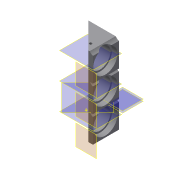
# Autodesk Inventor part: 30_Cube_Insert_Filter_Revolver_Filter_base
Saved by Autodesk Inventor 2019.4 (Build 234330000, 330)
## iProperties
Created: 2021-09-13
Part Number: 30_Cube_Insert_Filter_Revolver_Filter_base
Material: Generic
Document SubType Name: Modeling
Designer: diederichbenedict
Density: 1 g/cm^3
Appearance: Default
Mass: 6.97028 g
Surface Area: 48.8121 cm^2
Volume: 6.97028 cm^3
Author: diederichbenedict
Autodesk Inventor part; units mm, degrees
ref_plane "YZ Plane" through (0, 0, 0) normal (1, 0, 0) x (0, 1, 0)
ref_plane "XZ Plane" through (0, 0, 0) normal (0, 1, 0) x (-1, 0, 0)
ref_plane "XY Plane" through (0, 0, 0) normal (0, 0, 1) x (1, 0, 0)
ref_plane "Work Plane1" through (-34.3358, -34.38, 2.0699) normal (0, -1, 0) x (0.7071068, 0, -0.7071068)
ref_plane "Work Plane4" through (-9.5871, -34.38, 28.2329) normal (0, -1, 0) x (1, 0, 0)
ref_plane "Work Plane3" through (-9.5871, -32.38, 28.2329) normal (0, -1, 0) x (1, 0, 0)
sketch "Sketch1" plane through (-9.5871, -34.38, 28.2329) normal (0, -1, 0) x (1, 0, 0)
  line L0 (0.7071, -1.3185) -> (0.7071, -26.3185) construction
  line L1 (0.7071, -1.3185) -> (1.7071, -1.3185) construction
  line L2 (0.7071, -26.3185) -> (1.7071, -26.3185) construction
  line L3 (0.7071, -0.7071) -> (-26.8187, -28.2329)
  line L4 (-26.8187, -28.2329) -> (0.7071, -28.2329)
  line L5 (0.7071, -28.2329) -> (0.7071, -0.7071)
  line L6 (0.7071, -0.7071) -> (5.7071, -0.7071)
  line L7 (5.7071, -0.7071) -> (5.7071, -28.2329)
  line L8 (5.7071, -28.2329) -> (0.7071, -28.2329)
  line L9 (0.7071, -0.7071) -> (5.7071, -0.7071)
  line L10 (5.7071, -0.7071) -> (5.7071, 1.3671)
  line L11 (5.7071, 1.3671) -> (0.7071, 1.3671)
  line L12 (0.7071, 1.3671) -> (0.7071, -0.7071)
  line L13 (2.5336, 1.8671) -> (2.3871, 1.8671) projected
  line L14 (0.7071, -0.7071) -> (0.7071, -28.2329)
  line L15 (0.7071, -28.2329) -> (-26.8187, -28.2329)
  line L16 (-26.8187, -28.2329) -> (0.7071, -0.7071)
  point P0 (9.5871, -28.2329)
  dimension "d1" = 5
  dimension "d3" = 0.5
  constraints: 30 end point, 5 perpendicular, 3 equal length, 3 horizontal, 2 point on line, 2 other
  measures "d1" distance of L5.end L6.end
  measures "d3" distance between parallel lines of L11 L13
extrude "Extrusion1" add sketch "Sketch1" against normal blind 28 contours L5 L4 L3 | L6 L7 L8 L5
sketch "Sketch5" plane through (-3.88, -34.38, 0) normal (0, 0, -1) x (-1, 0, 0)
  line L0 (0, 0) -> (32.5258, 0) projected
  line L1 (32.5258, 0) -> (32.5258, 28) projected
  line L2 (0, 28) -> (32.5258, 28) projected
  line L3 (0, 0) -> (0, 28) projected
  line L4 (30.8258, 1.7) -> (1.7, 1.7)
  line L5 (1.7, 1.7) -> (1.7, 26.3)
  line L6 (1.7, 26.3) -> (30.8258, 26.3)
  line L7 (30.8258, 26.3) -> (30.8258, 1.7)
  circle A0 centre (24.5258, 1.7) radius 1.4
  circle A1 centre (8, 1.7) radius 1.4
  circle A2 centre (8, 26.3) radius 1.4
  circle A3 centre (24.5258, 26.3) radius 1.4
  point P0 (-3.88, 34.38)
  dimension "d19" = 1.7
  dimension "d20" = 2.8
  dimension "d21" = 2.8
  dimension "d22" = 2.8
  dimension "d23" = 2.8
  dimension "d24" = 8
  dimension "d25" = 8
  dimension "d26" = 8
  dimension "d27" = 8
  constraints: 8 end point, 4 centre point, 4 point on line, 3 other
  measures "d19" distance between parallel lines of L0 L4
  measures "d20" diameter of A0
  measures "d21" diameter of A1
  measures "d22" diameter of A2
  measures "d23" diameter of A3
  measures "d24" distance from line of A0.centre L1
  measures "d25" distance from line of A1.centre L3
  measures "d26" distance from line of L3 A2.centre
  measures "d27" distance from line of L1 A3.centre
extrude "Extrusion5" cut sketch "Sketch5" against normal blind 5 contours A0 L4 | L4 A0 | A3 L6 | L6 A3 | A1 L4 | L4 A1 | A2 L6 | L6 A2
sketch "Sketch6" plane through (-3.88, -34.38, 27.5258) normal (0, 0, 1) x (1, 0, 0)
  circle A0 centre (3.88, 34.38) radius 9.7565
  line L0 (0, 0) -> (-32.5258, 0) projected
  line L1 (-32.6288, 1.8364) -> (-30.8098, -0.0697)
  line L2 (-30.8098, -0.0697) -> (-32.6979, -0.0697)
  line L3 (-32.5258, 0) -> (-32.5258, 28) projected
  line L4 (-32.6979, -0.0697) -> (-32.6288, 1.8364)
  arc A1 (-42.4624, 56.6545) -> (-4.6674, -8.8083) centre (3.9, 39.78) ccw projected
  arc A2 (-37.2068, 12.4952) -> (-23.0987, -1.5152) centre (3.9, 39.78) ccw
  line L5 (-23.0987, -1.5152) -> (-43.2789, -2.9971)
  line L6 (-43.2789, -2.9971) -> (-37.2068, 12.4952)
  line L7 (0, 25.4281) -> (0, 28)
  line L8 (0, 28) -> (-3.5014, 28)
  line L9 (-5, 28) -> (0, 28) projected
  point P0 (-32.5258, 1.5)
  point P1 (-32.5258, 26.5)
  point P2 (-25.2852, 0)
  point P3 (-32.5258, 6.5026)
  constraints: 14 end point, 8 point on circle, 3 point on line, 2 centre point, 1 coincident, 1 concentric, 1 perpendicular
extrude "Extrusion6" cut sketch "Sketch6" against normal through all contours L8 L7 A0 picked at (-1.9896, 27.6569)
ref_plane "Work Plane5" through (-9.5871, -20.38, 28.2329) normal (0, -1, 0) x (1, 0, 0)
ref_plane "Work Plane6" through (-11.0013, -34.38, 27.5258) normal (0, 0, 1) x (1, 0, 0)
sketch "Sketch4" plane through (-3.88, -34.38, 27.5258) normal (1, 0, 0) x (0, 0, -1)
  circle A0 centre (13.1114, 14.5) radius 12.5 projected
  circle A1 centre (13.1114, 14.5) radius 11
  point P0 (27.5258, 34.38)
  dimension "d13" = 22
  constraints: 1 centre point, 1 coincident
  measures "d13" diameter of A1
extrude "Extrusion4" cut sketch "Sketch4" against normal through all contours A1
sketch "Sketch9" plane through (-8.88, -34.38, 27.5258) normal (-0.7071068, 0, 0.7071068) x (0.7071068, 0, 0.7071068)
  ellipse E0 centre (-18.5424, 14.5) end of major axis (-2.986, 14.5) minor radius 11 projected
  line L0 (-18.5424, 3.5) -> (-0.2544, 3.5)
  line L1 (-0.2544, 3.5) -> (-0.2544, 25.7594)
  line L2 (-0.2544, 25.7594) -> (-18.5424, 25.7594)
  line L3 (-18.5424, 25.7594) -> (-18.5424, 3.5)
  point P0 (-13.1846, 34.38)
  constraints: 8 end point, 2 parallel, 1 horizontal, 1 perpendicular, 1 vertical alignment, 1 other
extrude "Extrusion9" add sketch "Sketch9" against normal blind 3
sketch "Sketch10" plane through (-8.88, -34.38, 27.5258) normal (-0.7071068, 0, 0.7071068) x (0.7071068, 0, 0.7071068)
  ellipse E0 centre (-18.5424, 14.5) end of major axis (-2.986, 14.5) minor radius 11 (-18.5424, 3.5) -> (-18.5424, 25.5) ccw projected
  circle A0 centre (-18.5424, 14.5) radius 12.75
  point P0 (-13.1846, 34.38)
  dimension "d41" = 25.5
  constraints: 1 centre point, 1 coincident, 1 other
  measures "d41" diameter of A0
extrude "Extrusion10" cut sketch "Sketch10" against normal blind 1 contours A0
sketch "Sketch3" plane through (-3.88, -34.38, 27.5258) normal (1, 0, 0) x (0, 0, -1)
  circle A0 centre (13.1114, 14.5) radius 12.5 projected
  circle A1 centre (13.1114, 14.5) radius 12.8
  point P0 (27.5258, 34.38)
  dimension "d10" = 25.6
  constraints: 1 centre point, 1 coincident
  measures "d10" diameter of A1
extrude "Extrusion3" cut sketch "Sketch3" against normal blind 5.6 contours A0 | A1
sketch "Sketch11" plane through (-9.48, -34.38, 27.5258) normal (1, 0, 0) x (0, 0, -1)
  arc A0 (4.8426, 7.2455) -> (4.8426, 21.7545) centre (13.1114, 14.5) ccw projected
  circle A1 centre (13.1114, 14.5) radius 11
  point P0 (27.5258, 34.38)
  constraints: 1 centre point, 1 coincident, 1 concentric
extrude "Extrusion11" cut sketch "Sketch11" along normal up to surface surface through (-21.2843, -19.88, 13.7073) normal (-0.7071068, 0, 0.7071068)
sketch "Sketch12" plane through (-9.5871, -34.38, 28.2329) normal (0, -1, 0) x (1, 0, 0)
  line L0 (5.7071, -28.2329) -> (-26.8187, -28.2329) projected
  line L1 (5.7071, -0.7071) -> (5.7071, -28.2329) projected
  line L2 (0.7071, -0.7071) -> (5.7071, -0.7071) projected
  line L3 (-26.8187, -28.2329) -> (0.7071, -0.7071) projected
  circle A0 centre (-4.2596, -8.3038) radius 1.4
  point P0 (9.5871, -28.2329)
  dimension "d46" = 2.8
  constraints: 1 centre point
  measures "d46" diameter of A0
extrude "Extrusion12" cut sketch "Sketch12" against normal through all contours A0
sketch "Sketch13" plane through (-8.88, -34.38, 27.5258) normal (-0.7071068, 0, 0.7071068) x (0.7071068, 0, 0.7071068)
  ellipse E0 centre (-18.5424, 14.5) end of major axis (-0.4404, 14.5) minor radius 12.8 (-0.8485, 11.7974) -> (-0.8485, 17.2026) ccw projected
  line L0 (-0.8485, 11.7974) -> (-0.8485, 17.2026) projected
  circle A0 centre (-18.5424, 14.5) radius 12.75 projected
  line L1 (-38.9273, 0) -> (0, 0) projected
  line L2 (0, 0) -> (0, 28) projected
  line L3 (-38.9273, 28) -> (0, 28) projected
  line L4 (-38.9273, 0) -> (-38.9273, 28) projected
  circle A1 centre (-33.5424, 14.5) radius 1.45
  circle A2 centre (-4.0424, 6) radius 1.45
  circle A3 centre (-4.0424, 23) radius 1.45
  point P0 (-13.1846, 34.38)
  dimension "d49" = 2.9
  dimension "d50" = 2.9
  dimension "d51" = 2.9
  dimension "d52" = 15
  dimension "d53" = 0
  dimension "d54" = 8.5
  dimension "d55" = 8.5
  dimension "d56" = 14.5
  dimension "d57" = 0
  constraints: 3 centre point, 1 other
  measures "d49" diameter of A1
  measures "d50" diameter of A2
  measures "d51" diameter of A3
  measures "d52" distance of A1.centre point (-18.542, 14.5)
  measures "d53" vertical distance of A1.centre point (-18.542, 14.5)
  measures "d54" vertical distance of point (-18.542, 14.5) A3.centre
  measures "d55" vertical distance of point (-18.542, 14.5) A2.centre
  measures "d56" horizontal distance of point (-18.542, 14.5) A3.centre
  measures "d57" horizontal distance of A3.centre A2.centre
extrude "Extrusion13" cut sketch "Sketch13" against normal blind 10 contours A1 | A2 | A3
pattern_linear "Rectangular Pattern1" count 3 spacing 28 along (0, 1, 0) of "Extrusion1", "Extrusion5", "Extrusion6", "Extrusion4", "Extrusion9", "Extrusion10", "Extrusion3", "Extrusion11", "Extrusion12", "Extrusion13" first direction both ways yes
ref_plane "Work Plane2" through (41.82, -7.88, -4) normal (0, -1, 0) x (1, 0, 0)
ref_plane "Work Plane7" through (-11.0013, -6.38, 27.5258) normal (0, 0, 1) x (1, 0, 0)
ref_plane "Work Plane8" through (-11.0013, -62.38, 27.5258) normal (0, 0, 1) x (1, 0, 0)
ref_plane "Work Plane9" through (-9.5871, 7.62, 28.2329) normal (0, -1, 0) x (1, 0, 0)
ref_plane "Work Plane10" through (-9.5871, -48.38, 28.2329) normal (0, -1, 0) x (1, 0, 0)
body "Solid1"
